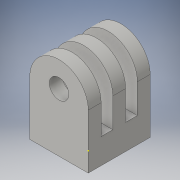
# Autodesk Inventor part: gopro_base
Saved by Autodesk Inventor 2016 (Build 200138000, 138)
## iProperties
Created: 2015-08-22
Part Number: gopro_base
Material: Generic
Document SubType Name: Modeling
Designer: Tyler
Density: 1 g/cm^3
Appearance: Default
Author: Tyler
Autodesk Inventor part; units mm, degrees
ref_plane "YZ Plane" through (0, 0, 0) normal (1, 0, 0) x (0, 1, 0)
ref_plane "XZ Plane" through (0, 0, 0) normal (0, 1, 0) x (-1, 0, 0)
ref_plane "XY Plane" through (0, 0, 0) normal (0, 0, 1) x (1, 0, 0)
sketch "Sketch4" plane through (0, 0, 0) normal (0, 0, 1) x (1, 0, 0)
  line L0 (-10.5, 0) -> (10.5, 0) projected
  line L1 (0, -3.3) -> (0, 19.8) projected
  line L2 (-7.5, 0) -> (7.5, 0)
  line L3 (7.5, 0) -> (7.5, 16.5)
  line L4 (7.5, 16.5) -> (-7.5, 16.5)
  line L5 (-7.5, 16.5) -> (-7.5, 0)
  circle A0 centre (0, 10) radius 2.5
  point P0 (0, 0)
  dimension "d0" = 7.5
  dimension "d1" = 7.5
  dimension "d2" = 16.5
  dimension "d3" = 5
  dimension "d4" = 6.5
  constraints: 8 end point, 2 parallel, 2 point on line, 1 centre point, 1 horizontal, 1 perpendicular
  measures "d0" distance between parallel lines of L1 L5
  measures "d1" distance between parallel lines of L1 L3
  measures "d2" distance between parallel lines of L4 L0
  measures "d3" diameter of A0
  measures "d4" distance from line of L4 A0.centre
extrude "Extrusion1" add sketch "Sketch4" against normal blind 15.9 contours L5 L4 L1 A0 L0 | L1 A0 L4 L3 L0
fillet "Fillet1" radius 7.5 2 edges at (7.5, 16.5, -7.95) (-7.5, 16.5, -7.95)
sketch "Sketch5" plane through (-7.5, 0, 0) normal (0, -1, 0) x (1, 0, 0)
  line L0 (0, 0) -> (0, -15.9) projected
  line L1 (15, 0) -> (15, -15.9) projected
  line L2 (0, 0) -> (15, 0)
  line L3 (15, 0) -> (15, -15.9)
  line L4 (15, -15.9) -> (0, -15.9)
  line L5 (0, -15.9) -> (0, 0)
  point P0 (7.5, 0)
  constraints: 8 end point, 2 parallel, 1 horizontal, 1 perpendicular
extrude "Extrusion2" add sketch "Sketch5" along normal blind 5
sketch "Sketch6" plane through (7.5, 9, 0) normal (1, 0, 0) x (0, 0, -1)
  point P0 (0, -9)
sketch "Sketch7" plane through (7.5, 9, 0) normal (1, 0, 0) x (0, 0, -1)
  line L0 (0, 0) -> (0, 7.5) projected
  line L1 (0, 7.5) -> (3.3, 7.5)
  line L2 (3.3, 7.5) -> (3.3, -7.5)
  line L3 (3.3, -7.5) -> (0, -7.5)
  line L4 (0, -7.5) -> (0, 7.5)
  line L5 (0, 7.5) -> (15.9, 7.5) projected
  line L6 (6.3, 7.5) -> (9.6, 7.5)
  line L7 (9.6, 7.5) -> (9.6, -7.5)
  line L8 (9.6, -7.5) -> (6.3, -7.5)
  line L9 (6.3, -7.5) -> (6.3, 7.5)
  line L10 (12.6, 7.5) -> (15.9, 7.5)
  line L11 (15.9, 7.5) -> (15.9, -7.5)
  line L12 (15.9, -7.5) -> (12.6, -7.5)
  line L13 (12.6, -7.5) -> (12.6, 7.5)
  line L14 (3.3, -7.5) -> (6.3, -7.5)
  line L15 (9.6, -7.5) -> (12.6, -7.5)
  line L16 (3.3, 7.5) -> (6.3, 7.5)
  line L17 (9.6, 7.5) -> (12.6, 7.5)
  point P0 (0, -9)
  dimension "d10" = 3.3
  dimension "d11" = 15
  dimension "d12" = 3
  dimension "d13" = 3.3
  dimension "d14" = 3
  dimension "d15" = 3.3
  constraints: 32 end point, 6 parallel, 4 horizontal, 4 point on line, 3 collinear, 3 perpendicular
  measures "d10" distance between parallel lines of L2 L0
  measures "d11" distance of L1.end L2.end
  measures "d12" distance between parallel lines of L9 L2
  measures "d13" distance between parallel lines of L7 L9
  measures "d14" distance between parallel lines of L7 L13
  measures "d15" distance between parallel lines of L11 L13
sketch "Sketch8" plane through (7.5, 9, 0) normal (1, 0, 0) x (0, 0, -1)
  line L0 (0, 7.5) -> (15.9, 7.5) projected
  line L1 (3.3, 7.5) -> (6.2995, 7.5)
  line L2 (6.2995, 7.5) -> (6.2995, -7.4999)
  line L3 (6.2995, -7.4999) -> (3.3, -7.4999)
  line L4 (3.3, -7.4999) -> (3.3, 7.5)
  line L5 (9.5994, 7.5) -> (12.5997, 7.5)
  line L6 (12.5997, 7.5) -> (12.5997, -7.4999)
  line L7 (12.5997, -7.4999) -> (9.5994, -7.4999)
  line L8 (9.5994, -7.4999) -> (9.5994, 7.5)
  point P0 (0, -9)
  constraints: 16 end point, 4 parallel, 3 point on line, 2 horizontal, 2 perpendicular
extrude "Extrusion3" cut sketch "Sketch7" against normal through all contours L5 L13 L15 L7
extrude "Extrusion4" cut sketch "Sketch8" against normal through all contours L0 L2 L3 L4
body "Solid1"
